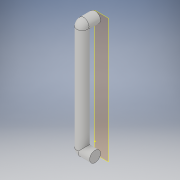
# Autodesk Inventor part: Exhaust 2
Saved by Autodesk Inventor 2019 (Build 230136000, 136)
## iProperties
Created: 2020-10-15
Part Number: Exhaust 2
Material: Generic
Document SubType Name: Modeling
Designer: nabee
Density: 1 g/cm^3
Appearance: Default
Author: nabee
Autodesk Inventor part; units mm, degrees
ref_plane "XZ Plane" through (0, 0, 0) normal (0, 1, 0) x (-1, 0, 0)
sketch "Sketch1" plane through (0, 0, 0) normal (0, 0, 1) x (1, 0, 0)
  point P0 (0, 0)
sketch "Sketch2" plane through (0, 0, 0) normal (1, 0, 0) x (0, 1, 0)
  point P0 (0, 0)
sketch "Sketch3" plane through (0, 0, 0) normal (0, 0, 1) x (1, 0, 0)
  point P0 (0, 0)
ref_plane "Work Plane1" through (60, 0, 0) normal (1, 0, 0) x (0, 1, 0)
sketch "Sketch4" plane through (60, 0, 0) normal (1, 0, 0) x (0, 1, 0)
  circle A0 centre (0, 0) radius 25
  dimension "d6" = 50
  constraints: 1 centre point, 1 coincident
  measures "d6" diameter of A0
ref_plane "Work Plane2" through (0, 0, -60) normal (0, 0, 1) x (1, 0, 0)
sketch "Sketch5" plane through (0, 0, -60) normal (0, 0, 1) x (1, 0, 0)
  point P0 (0, 0)
sketch3d "3D Sketch1"
  line L0 (60, 0, 0) -> (7, 0, 0)
  arc A0 (7, 0, 0) -> (0, 7, 0) centre (7, 7, 0) ccw
  line L1 (0, 7, 0) -> (0, 493, 0)
  arc A1 (0, 493, 0) -> (0, 500, -7) centre (0, 493, -7) ccw
  line L2 (0, 500, -7) -> (0, 500, -60)
  dimension "d0" = 500
  dimension "d1" = 60
  dimension "d2" = 60
  dimension "d8" = 7
  dimension "d9" = 7
sweep "Sweep1" add profiles "Sketch4" path "3D Sketch1"
body "Solid1"
